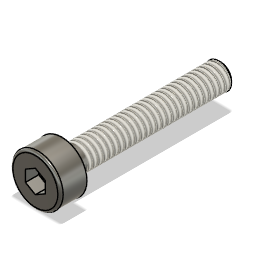
mmWave v4 (Autodesk Fusion 360 archive; units mm, degrees)
design "Hexagon Socket Head Cap Screw ISO 4762 - M2 x 12 Steel 4.6 Plain"
description: Hexagon Socket Head Cap Screw ISO 4762 - M2 x 12
part number: ISO 4762 - M2 x 12 Steel 4.6 Plain
Autodesk Fusion 360 part; units mm, degrees
sketch "Sketch1" plane through (0, 0, 0) normal (0, 1, 0) x (1, 0, 0)
  line L0 (-1, 0) -> (-1, 12)
  line L1 (-1, 12) -> (0, 12)
  line L2 (0, 12) -> (0, -2)
  line L3 (-1, 0) -> (-1.9, 0)
  line L4 (-1.9, 0) -> (-1.9, -2)
  line L5 (-1.9, -2) -> (0, -2)
  dimension "d9" = 2
  dimension "d66" = 3.8
  dimension "d106" = 2
  dimension "d107" = 12
  constraint perpendicular L0 L1
  constraint collinear origin L1.end L2.end
  constraint perpendicular L0 L3
  constraint coincident origin L3
  constraint vertical L0
  constraint vertical L2
  constraint parallel L2 L4
  constraint coincident L2 L5.end
  constraint perpendicular L2 L5
  measures "d106" distance of L3 L5
  measures "d107" distance of origin L1
revolve "Revolve1" add sketch "Sketch1" angle 360 about axis through (0, 0, -12) along (0, 0, 1)
ref_plane "WorkPlane1" through (0, 0, 2) normal (0, 0, 1) x (1, 0, 0)
sketch "Sketch6" plane through (0, 0, 2) normal (0, 0, 1) x (1, 0, 0)
  line L0 (-0.75, 0) -> (0.75, 0) construction
  line L1 (0, 0) -> (-0.75, 0.433)
  line L2 (-0.75, -0.433) -> (-0.75, 0.433)
  line L3 (-0.75, -0.433) -> (0, 0)
  dimension "d104" = 150
  dimension "d108" = 1.5
  constraint horizontal L0
  constraint midpoint L1.start L0
  constraint coincident L1.start L3.end
  constraint perpendicular L0 L2
  constraint midpoint L0.start L2
  constraint coincident L1.end L2.end
  measures "d104" angle of L0 L1
  measures "d108" distance of L0.end L2
extrude "Extrude1" cut sketch "Sketch6" against normal blind 1
pattern_circular "C-Pattern1" count 6 over 360 about axis through (0, 0, 1.75) along (0, 0, 1) of "Extrude1"
extrude "Extrude2" cut 1 faces at (0, 0.2887, 1) along direction (0, 0, -1) blind 1 draft -85
fillet "Fillet4" radius 0.2 1 edges at (-1.7714, 0.6871, 2)
thread "Thread3" "ISO Metric profile 2.0 M2x0.4 M2x0.4 6g" major diameter 1.9335 minor diameter 1.478 pitch 0.4 angle 60 resizes the face on face at (-0.9988, 0.0498, -4) from (0, 0, -1) to (0, 0, -12)
sketch "Sketch7" plane through (0, 0, 0) normal (0, 1, 0) x (1, 0, 0)
  line L0 (-1.02, 12) -> (-1.02, 11.8)
  line L1 (-1.02, 11.8) -> (-0.82, 12)
  line L2 (0, 12) -> (0, -2)
  line L3 (-1.02, 12) -> (0, 12)
  dimension "d101" = 45
  dimension "d112" = 0.2
  dimension "d113" = 1.02
  constraint coincident L2.start L3.end
  constraint perpendicular L2 L3
  constraint coincident L1.end L3
  constraint perpendicular L0 L3
  measures "d101" angle of L0 L1
  measures "d112" distance of L0.end L3
  measures "d113" distance of L0 L2.start
revolve "Revolve3" cut sketch "Sketch7" angle 360 about axis through (0, 0, 1.75) along (0, 0, 1)
equation "d9 = adsk_nomdia"
equation "adsk_nomlen = 12.00 mm"
equation "adsk_headh = 2.00 mm"
equation "adsk_headdia = 3.80 mm"
equation "adsk_nomdia = 2.00 mm"
equation "adsk_philwidth = 1.50 mm"
equation "d31 = -adsk_phildepth"
equation "adsk_phildepth = 1.00 mm"
equation "d66 = adsk_headdia"
equation "d71 = adsk_headh"
equation "d76 = -adsk_phildepth"
equation "adsk_thrlen = 11.00 mm"
equation "d86 = adsk_nomdia * 0.1"
equation "adsk_startang = 45.00 deg"
equation "d101 = adsk_startang"
equation "adsk_pitch1 = 0.40 mm"
equation "adsk_startlen = 0.20 mm"
equation "d106 = adsk_headh"
equation "d107 = adsk_nomlen"
equation "d108 = adsk_philwidth"
equation "d112 = adsk_startlen"
equation "d113 = adsk_nomdia * 0.51"
equation "d115 = min(adsk_thrlen; adsk_nomlen - 0.001 mm)"

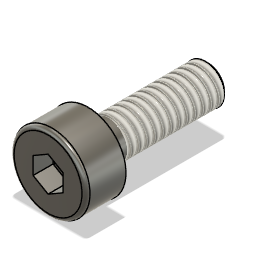
design "Hexagon Socket Head Cap Screw ISO 4762 - M2 x 6 Steel 4.6 Plain"
description: Hexagon Socket Head Cap Screw ISO 4762 - M2 x 6
part number: ISO 4762 - M2 x 6 Steel 4.6 Plain
Autodesk Fusion 360 part; units mm, degrees
sketch "Sketch1" plane through (0, 0, 0) normal (0, 1, 0) x (1, 0, 0)
  line L0 (-1, 0) -> (-1, 6)
  line L1 (-1, 6) -> (0, 6)
  line L2 (0, 6) -> (0, -2)
  line L3 (-1, 0) -> (-1.9, 0)
  line L4 (-1.9, 0) -> (-1.9, -2)
  line L5 (-1.9, -2) -> (0, -2)
  dimension "d9" = 2
  dimension "d66" = 3.8
  dimension "d106" = 2
  dimension "d107" = 6
  constraint perpendicular L0 L1
  constraint collinear origin L1.end L2.end
  constraint perpendicular L0 L3
  constraint coincident origin L3
  constraint vertical L0
  constraint vertical L2
  constraint parallel L2 L4
  constraint coincident L2 L5.end
  constraint perpendicular L2 L5
  measures "d106" distance of L3 L5
  measures "d107" distance of origin L1
revolve "Revolve1" add sketch "Sketch1" angle 360 about axis through (0, 0, -6) along (0, 0, 1)
ref_plane "WorkPlane1" through (0, 0, 2) normal (0, 0, 1) x (1, 0, 0)
sketch "Sketch6" plane through (0, 0, 2) normal (0, 0, 1) x (1, 0, 0)
  line L0 (-0.75, 0) -> (0.75, 0) construction
  line L1 (0, 0) -> (-0.75, 0.433)
  line L2 (-0.75, -0.433) -> (-0.75, 0.433)
  line L3 (-0.75, -0.433) -> (0, 0)
  dimension "d104" = 150
  dimension "d108" = 1.5
  constraint horizontal L0
  constraint midpoint L1.start L0
  constraint coincident L1.start L3.end
  constraint perpendicular L0 L2
  constraint midpoint L0.start L2
  constraint coincident L1.end L2.end
  measures "d104" angle of L0 L1
  measures "d108" distance of L0.end L2
extrude "Extrude1" cut sketch "Sketch6" against normal blind 1
pattern_circular "C-Pattern1" count 6 over 360 about axis through (0, 0, 1.75) along (0, 0, 1) of "Extrude1"
extrude "Extrude2" cut 1 faces at (0, 0.2887, 1) along direction (0, 0, -1) blind 1 draft -85
fillet "Fillet4" radius 0.2 1 edges at (-1.7714, 0.6871, 2)
thread "Thread3" "ISO Metric profile 2.0 M2x0.4 M2x0.4 6g" major diameter 1.9335 minor diameter 1.478 pitch 0.4 angle 60 resizes the face on face at (-0.9988, 0.0498, -4) from (0, 0, -1) to (0, 0, -6)
sketch "Sketch7" plane through (0, 0, 0) normal (0, 1, 0) x (1, 0, 0)
  line L0 (-1.02, 6) -> (-1.02, 5.8)
  line L1 (-1.02, 5.8) -> (-0.82, 6)
  line L2 (0, 6) -> (0, -2)
  line L3 (-1.02, 6) -> (0, 6)
  dimension "d101" = 45
  dimension "d112" = 0.2
  dimension "d113" = 1.02
  constraint coincident L2.start L3.end
  constraint perpendicular L2 L3
  constraint coincident L1.end L3
  constraint perpendicular L0 L3
  measures "d101" angle of L0 L1
  measures "d112" distance of L0.end L3
  measures "d113" distance of L0 L2.start
revolve "Revolve3" cut sketch "Sketch7" angle 360 about axis through (0, 0, 1.75) along (0, 0, 1)
equation "d9 = adsk_nomdia"
equation "adsk_nomlen = 6.00 mm"
equation "adsk_headh = 2.00 mm"
equation "adsk_headdia = 3.80 mm"
equation "adsk_nomdia = 2.00 mm"
equation "adsk_philwidth = 1.50 mm"
equation "d31 = -adsk_phildepth"
equation "adsk_phildepth = 1.00 mm"
equation "d66 = adsk_headdia"
equation "d71 = adsk_headh"
equation "d76 = -adsk_phildepth"
equation "adsk_thrlen = 5.00 mm"
equation "d86 = adsk_nomdia * 0.1"
equation "adsk_startang = 45.00 deg"
equation "d101 = adsk_startang"
equation "adsk_pitch1 = 0.40 mm"
equation "adsk_startlen = 0.20 mm"
equation "d106 = adsk_headh"
equation "d107 = adsk_nomlen"
equation "d108 = adsk_philwidth"
equation "d112 = adsk_startlen"
equation "d113 = adsk_nomdia * 0.51"
equation "d115 = min(adsk_thrlen; adsk_nomlen - 0.001 mm)"

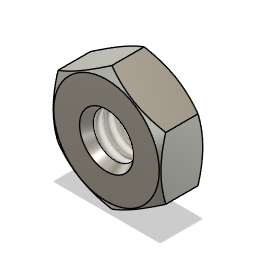
design "Hexagon Regular Nut ISO 4032 - M2 Steel 6 Plain"
description: Hexagon Regular Nut ISO 4032 - M2
part number: ISO 4032 - M2 Steel 6 Plain
Autodesk Fusion 360 part; units mm, degrees
sketch "Sketch1" plane through (0, 0, 0) normal (0, 1, 0) x (1, 0, 0)
  line L0 (0, 0) -> (0, -1.6)
  line L1 (-1, 0) -> (-1.96, 0)
  line L2 (-1.96, 0) -> (-2.31, -0.2021)
  line L3 (-2.31, -0.2021) -> (-2.31, -1.3979)
  line L4 (-2.31, -1.3979) -> (-1.96, -1.6)
  line L5 (-1.96, -1.6) -> (-1, -1.6)
  line L6 (-1, -1.6) -> (-1, 0)
  dimension "d121" = 2
  dimension "d122" = 30
  dimension "d123" = 30
  dimension "d128" = 4.62
  dimension "d172" = 3.92
  dimension "d176" = 1.6
  constraint vertical L0
  constraint coincident L0 L0.end
  constraint coincident origin L0
  constraint horizontal L1
  constraint perpendicular L1 L3
  constraint perpendicular L3 L5
  constraint perpendicular L5 L6
  constraint coincident L0.start L1
  constraint coincident L0.start origin
  constraint coincident L0.end L5
  constraint vertical L1.end L4.end
  measures "d122" angle of L1 L2
  measures "d123" angle of L4 L5
  measures "d176" distance of L1.start L5
revolve "Revolve1" add sketch "Sketch1" angle 360 about axis through (0, 0, 0) along (0, 0, 1)
sketch "Sketch8" plane through (0, 0, 1.6) normal (0, 0, 1) x (1, 0, 0)
  line L0 (0, 0) -> (-4, 0) construction
  line L1 (-2, -1.1559) -> (-2, 1.1559)
  circle A0 centre (0, 0) radius 1
  circle A1 centre (0, 0) radius 2.31
  dimension "d114" = 2
  constraint horizontal L0
  constraint perpendicular L0 L1
  constraint midpoint L0 L1
  constraint coincident L0.start A0.centre
  constraint coincident L1.end A1
  measures "d114" distance of L0.start L1
extrude "Extrude5" cut sketch "Sketch8" against normal blind 1.6 contours L1 A1 picked at (-2.05, 0.2815)
pattern_circular "C-Pattern2" count 6 over 360 about axis through (0, 0, 1.75) along (0, 0, 1) of "Extrude5"
thread "Thread3" "ISO Metric profile 2.0 M2x0.4 M2x0.4 6H" major diameter 2.074 minor diameter 1.623 pitch 0.4 angle 60 resizes the face on face at (-0.9988, 0.0498, 1.0667)
sketch "Sketch12" plane through (0, 0, 0) normal (0, 1, 0) x (1, 0, 0)
  line L0 (0.8115, -1.6) -> (-0.8115, -1.6)
  line L1 (1.96, -1.6) -> (-1.96, -1.6)
  line L2 (1.96, 0) -> (-1.96, 0)
  line L3 (0.8115, 0) -> (-0.8115, 0)
  line L4 (-1, 0) -> (0, 0)
  line L5 (-0.5381, -0.8) -> (-1, 0)
  line L6 (-1, -1.6) -> (0, -1.6)
  line L7 (-0.5381, -0.8) -> (-1, -1.6)
  line L8 (0, 0) -> (0, -1.6)
  dimension "d165" = 60
  dimension "d169" = 60
  dimension "d177" = 1
  constraint horizontal L4
  constraint collinear L1 L6
  constraint coincident L5.start L7.start
  constraint vertical L4.start L6.start
  constraint coincident L1 L6.end
  constraint coincident L6.end L8.end
  constraint coincident L4.end L8.start
  measures "d165" angle of L2 L5
  measures "d169" angle of L6 L7
  measures "d177" distance of L4.start L8
revolve "Revolve3" cut sketch "Sketch12" angle 360 about axis through (0, 0, 1.75) along (0, 0, 1)
equation "adsk_nheig = 1.60 mm"
equation "adsk_maxdia = 4.62 mm"
equation "adsk_nomdia = 2.00 mm"
equation "d89 = -adsk_nheig"
equation "adsk_waflat = 4.00 mm"
equation "d114 = adsk_waflat / 2"
equation "adsk_chamang1 = 30.00 deg"
equation "adsk_chamang2 = 30.00 deg"
equation "d121 = adsk_nomdia"
equation "d122 = adsk_chamang1"
equation "d123 = adsk_chamang2"
equation "d128 = adsk_maxdia"
equation "d163 = adsk_nheig"
equation "adsk_beardia = 3.92 mm"
equation "d172 = adsk_beardia"
equation "d176 = adsk_nheig"
equation "d177 = adsk_nomdia * 0.5"
